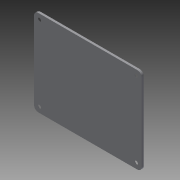
# Autodesk Inventor part: WYKONAWCY
Saved by Autodesk Inventor 2014 (Build 180170000, 170)
## iProperties
Created: 2017-04-20
Part Number: WYKONAWCY
Material: Ogólny
Document SubType Name: Modeling
Designer: hpdc7700
Density: 1 g/cm^3
Appearance: Domyślna
Author: hpdc7700
Autodesk Inventor part; units mm, degrees
(part 1 of 3)
ref_plane "YZ Plane" through (0, 0, 0) normal (1, 0, 0) x (0, 1, 0)
ref_plane "XZ Plane" through (0, 0, 0) normal (0, 1, 0) x (-1, 0, 0)
ref_plane "XY Plane" through (0, 0, 0) normal (0, 0, 1) x (1, 0, 0)
sketch "Szkic1" plane through (0, 0, 0) normal (0, 1, 0) x (-1, 0, 0)
  line L0 (-50, -40) -> (50, -40)
  line L1 (50, -40) -> (50, 40)
  line L2 (50, 40) -> (-50, 40)
  line L3 (-50, 40) -> (-50, -40)
  line L4 (-50, -40) -> (50, 40) construction
  line L5 (50, -40) -> (-50, 40) construction
  point P0 (0, 0)
  dimension "d0" = 100
  dimension "d1" = 80
  constraints: 12 end point, 2 midpoint, 2 parallel, 1 horizontal, 1 perpendicular
  measures "d0" distance of L2.end L1.end
  measures "d1" distance of L1.end L0.end
extrude "Wyciągnięcie proste1" add sketch "Szkic1" along normal blind 2
sketch "Szkic2" plane through (0, 2, 0) normal (0, 1, 0) x (1, 0, 0)
  line L0 (-46.7747, 36.4699) -> (46.5954, 36.4699) construction
  line L1 (46.5954, 36.4699) -> (46.5954, -36.8283) construction
  line L2 (46.5954, -36.8283) -> (-46.7747, -36.8283) construction
  line L3 (-46.7747, -36.8283) -> (-46.7747, 36.4699) construction
  line L4 (-33.4162, 27.0179) -> (-34.6723, 22.0179)
  line L5 (-34.6723, 22.0179) -> (-35.4178, 22.0179)
  line L6 (-35.4178, 22.0179) -> (-36.4348, 26.167)
  line L7 (-36.4348, 26.167) -> (-37.4235, 22.0179)
  line L8 (-37.4235, 22.0179) -> (-38.1609, 22.0179)
  line L9 (-38.1609, 22.0179) -> (-39.4373, 27.0179)
  line L10 (-39.4373, 27.0179) -> (-38.7525, 27.0179)
  line L11 (-38.7525, 27.0179) -> (-37.7476, 22.8728)
  line L12 (-37.7476, 22.8728) -> (-36.7509, 27.0179)
  line L13 (-36.7509, 27.0179) -> (-36.0742, 27.0179)
  line L14 (-36.0742, 27.0179) -> (-35.0693, 22.8242)
  line L15 (-35.0693, 22.8242) -> (-34.0685, 27.0179)
  line L16 (-34.0685, 27.0179) -> (-33.4162, 27.0179)
  line L17 (-29.3198, 27.0179) -> (-31.0094, 24.2302)
  line L18 (-31.0094, 24.2302) -> (-31.0094, 22.0179)
  line L19 (-31.0094, 22.0179) -> (-31.6739, 22.0179)
  line L20 (-31.6739, 22.0179) -> (-31.6739, 24.1613)
  line L21 (-31.6739, 24.1613) -> (-33.3635, 27.0179)
  line L22 (-33.3635, 27.0179) -> (-32.6261, 27.0179)
  line L23 (-32.6261, 27.0179) -> (-31.3376, 24.8177)
  line L24 (-31.3376, 24.8177) -> (-30.0248, 27.0179)
  line L25 (-30.0248, 27.0179) -> (-29.3198, 27.0179)
  line L26 (-25.2112, 22.0179) -> (-26.0742, 22.0179)
  line L27 (-26.0742, 22.0179) -> (-27.9016, 24.3437)
  line L28 (-27.9016, 24.3437) -> (-28.1933, 24.0155)
  line L29 (-28.1933, 24.0155) -> (-28.1933, 22.0179)
  line L30 (-28.1933, 22.0179) -> (-28.8578, 22.0179)
  line L31 (-28.8578, 22.0179) -> (-28.8578, 27.0179)
  line L32 (-28.8578, 27.0179) -> (-28.1933, 27.0179)
  line L33 (-28.1933, 27.0179) -> (-28.1933, 24.7205)
  line L34 (-28.1933, 24.7205) -> (-26.1431, 27.0179)
  line L35 (-26.1431, 27.0179) -> (-25.3327, 27.0179)
  line L36 (-25.3327, 27.0179) -> (-27.4032, 24.7853)
  line L37 (-27.4032, 24.7853) -> (-25.2112, 22.0179)
  spline S0 degree 2 poles (-21.2768, 26.4466) (-20.9932, 26.1143) (-20.6771, 25.1419) (-20.6771, 24.5179) knots 0 0 0 1 2 2 2
  spline S1 degree 2 poles (-20.6771, 24.5179) (-20.6771, 23.9101) (-20.9851, 22.9255) (-21.2768, 22.5933) knots 0 0 0 1 2 2 2
  spline S2 degree 2 poles (-21.2768, 22.5933) (-21.5847, 22.2448) (-22.3992, 21.9125) (-22.8894, 21.9125) knots 0 0 0 1 2 2 2
  spline S3 degree 2 poles (-22.8894, 21.9125) (-23.3959, 21.9125) (-24.2063, 22.257) (-24.5021, 22.5933) knots 0 0 0 1 2 2 2
  spline S4 degree 2 poles (-24.5021, 22.5933) (-24.7898, 22.9255) (-25.0977, 23.902) (-25.0977, 24.5179) knots 0 0 0 1 2 2 2
  spline S5 degree 2 poles (-25.0977, 24.5179) (-25.0977, 25.1459) (-24.7857, 26.1022) (-24.498, 26.4466) knots 0 0 0 1 2 2 2
  spline S6 degree 2 poles (-24.498, 26.4466) (-24.2063, 26.7788) (-23.3919, 27.1232) (-22.8894, 27.1232) knots 0 0 0 1 2 2 2
  spline S7 degree 2 poles (-22.8894, 27.1232) (-22.3789, 27.1232) (-21.5604, 26.7667) (-21.2768, 26.4466) knots 0 0 0 1 2 2 2
  spline S8 degree 2 poles (-21.37, 24.5179) (-21.37, 25.0122) (-21.5847, 25.778) (-21.7792, 26.0292) knots 0 0 0 1 2 2 2
  spline S9 degree 2 poles (-21.7792, 26.0292) (-21.9778, 26.2886) (-22.5369, 26.5479) (-22.8854, 26.5479) knots 0 0 0 1 2 2 2
  spline S10 degree 2 poles (-22.8854, 26.5479) (-23.246, 26.5479) (-23.789, 26.2967) (-23.9956, 26.0292) knots 0 0 0 1 2 2 2
  spline S11 degree 2 poles (-23.9956, 26.0292) (-24.1941, 25.774) (-24.4048, 25.0041) (-24.4048, 24.5179) knots 0 0 0 1 2 2 2
  spline S12 degree 2 poles (-24.4048, 24.5179) (-24.4048, 23.5333) (-23.5783, 22.4879) (-22.8854, 22.4879) knots 0 0 0 1 2 2 2
  spline S13 degree 2 poles (-22.8854, 22.4879) (-22.1925, 22.4879) (-21.37, 23.5333) (-21.37, 24.5179) knots 0 0 0 1 2 2 2
  line L38 (-16.37, 22.0179) -> (-17.1155, 22.0179)
  line L39 (-17.1155, 22.0179) -> (-19.3279, 26.3291)
  line L40 (-19.3279, 26.3291) -> (-19.3279, 22.0179)
  line L41 (-19.3279, 22.0179) -> (-19.9478, 22.0179)
  line L42 (-19.9478, 22.0179) -> (-19.9478, 27.0179)
  line L43 (-19.9478, 27.0179) -> (-19.0037, 27.0179)
  line L44 (-19.0037, 27.0179) -> (-16.9899, 23.0592)
  line L45 (-16.9899, 23.0592) -> (-16.9899, 27.0179)
  line L46 (-16.9899, 27.0179) -> (-16.37, 27.0179)
  line L47 (-16.37, 27.0179) -> (-16.37, 22.0179)
  line L48 (-15.8959, 22.0179) -> (-14.2104, 27.0179)
  line L49 (-14.2104, 27.0179) -> (-13.3919, 27.0179)
  line L50 (-13.3919, 27.0179) -> (-11.7063, 22.0179)
  line L51 (-11.7063, 22.0179) -> (-12.4073, 22.0179)
  line L52 (-12.4073, 22.0179) -> (-12.8611, 23.4158)
  line L53 (-12.8611, 23.4158) -> (-14.7695, 23.4158)
  line L54 (-14.7695, 23.4158) -> (-15.2233, 22.0179)
  line L55 (-15.2233, 22.0179) -> (-15.8959, 22.0179)
  line L56 (-13.0434, 23.983) -> (-13.8173, 26.3372)
  line L57 (-13.8173, 26.3372) -> (-14.5872, 23.983)
  line L58 (-14.5872, 23.983) -> (-13.0434, 23.983)
  line L59 (-5.6285, 27.0179) -> (-6.8846, 22.0179)
  line L60 (-6.8846, 22.0179) -> (-7.6301, 22.0179)
  line L61 (-7.6301, 22.0179) -> (-8.6471, 26.167)
  line L62 (-8.6471, 26.167) -> (-9.6358, 22.0179)
  line L63 (-9.6358, 22.0179) -> (-10.3732, 22.0179)
  line L64 (-10.3732, 22.0179) -> (-11.6496, 27.0179)
  line L65 (-11.6496, 27.0179) -> (-10.9648, 27.0179)
  line L66 (-10.9648, 27.0179) -> (-9.9599, 22.8728)
  line L67 (-9.9599, 22.8728) -> (-8.9632, 27.0179)
  line L68 (-8.9632, 27.0179) -> (-8.2865, 27.0179)
  line L69 (-8.2865, 27.0179) -> (-7.2817, 22.8242)
  line L70 (-7.2817, 22.8242) -> (-6.2809, 27.0179)
  line L71 (-6.2809, 27.0179) -> (-5.6285, 27.0179)
  spline S14 degree 2 poles (-3.0799, 21.9288) (-3.5661, 21.9288) (-4.3886, 22.257) (-4.6885, 22.5852) knots 0 0 0 1 2 2 2
  spline S15 degree 2 poles (-4.6885, 22.5852) (-4.9883, 22.9093) (-5.3165, 23.8817) (-5.3165, 24.5138) knots 0 0 0 1 2 2 2
  spline S16 degree 2 poles (-5.3165, 24.5138) (-5.3165, 25.1419) (-4.9964, 26.0738) (-4.6925, 26.4182) knots 0 0 0 1 2 2 2
  spline S17 degree 2 poles (-4.6925, 26.4182) (-4.3927, 26.7545) (-3.5742, 27.107) (-3.0677, 27.107) knots 0 0 0 1 2 2 2
  spline S18 degree 2 poles (-3.0677, 27.107) (-2.8165, 27.107) (-2.3749, 27.0341) (-2.1885, 26.9774) knots 0 0 0 1 2 2 2
  spline S19 degree 2 poles (-2.1885, 26.9774) (-2.0264, 26.9247) (-1.6901, 26.7748) (-1.524, 26.6856) knots 0 0 0 1 2 2 2
  line L72 (-1.524, 26.6856) -> (-1.524, 25.8834)
  line L73 (-1.524, 25.8834) -> (-1.5766, 25.8834)
  spline S20 degree 2 poles (-1.5766, 25.8834) (-1.6658, 25.9644) (-1.9413, 26.1913) (-2.1398, 26.3007) knots 0 0 0 1 2 2 2
  spline S21 degree 2 poles (-2.1398, 26.3007) (-2.3303, 26.4061) (-2.78, 26.5398) (-3.0718, 26.5398) knots 0 0 0 1 2 2 2
  spline S22 degree 2 poles (-3.0718, 26.5398) (-3.3919, 26.5398) (-3.9632, 26.2764) (-4.1779, 26.0252) knots 0 0 0 1 2 2 2
  spline S23 degree 2 poles (-4.1779, 26.0252) (-4.3886, 25.7699) (-4.6236, 24.996) (-4.6236, 24.5138) knots 0 0 0 1 2 2 2
  spline S24 degree 2 poles (-4.6236, 24.5138) (-4.6236, 23.9993) (-4.3765, 23.2578) (-4.1617, 23.0025) knots 0 0 0 1 2 2 2
  spline S25 degree 2 poles (-4.1617, 23.0025) (-3.951, 22.7553) (-3.3878, 22.5041) (-3.0718, 22.5041) knots 0 0 0 1 2 2 2
  spline S26 degree 2 poles (-3.0718, 22.5041) (-2.7841, 22.5041) (-2.2938, 22.6459) (-2.1034, 22.7513) knots 0 0 0 1 2 2 2
  spline S27 degree 2 poles (-2.1034, 22.7513) (-1.921, 22.8566) (-1.6496, 23.0754) (-1.5726, 23.1524) knots 0 0 0 1 2 2 2
  line L74 (-1.5726, 23.1524) -> (-1.524, 23.1524)
  line L75 (-1.524, 23.1524) -> (-1.524, 22.3582)
  spline S28 degree 2 poles (-1.524, 22.3582) (-1.6901, 22.2813) (-1.9818, 22.1394) (-2.1885, 22.0746) knots 0 0 0 1 2 2 2
  spline S29 degree 2 poles (-2.1885, 22.0746) (-2.4073, 22.0017) (-2.78, 21.9288) (-3.0799, 21.9288) knots 0 0 0 1 2 2 2
  line L76 (2.5968, 27.0179) -> (0.9072, 24.2302)
  line L77 (0.9072, 24.2302) -> (0.9072, 22.0179)
  line L78 (0.9072, 22.0179) -> (0.2426, 22.0179)
  line L79 (0.2426, 22.0179) -> (0.2426, 24.1613)
  line L80 (0.2426, 24.1613) -> (-1.447, 27.0179)
  line L81 (-1.447, 27.0179) -> (-0.7095, 27.0179)
  line L82 (-0.7095, 27.0179) -> (0.579, 24.8177)
  line L83 (0.579, 24.8177) -> (1.8918, 27.0179)
  line L84 (1.8918, 27.0179) -> (2.5968, 27.0179)
  spline S30 degree 2 poles (8.3666, 25.5106) (8.3666, 25.1864) (8.1357, 24.603) (7.929, 24.4004) knots 0 0 0 1 2 2 2
  spline S31 degree 2 poles (7.929, 24.4004) (7.6697, 24.1451) (6.9687, 23.8817) (6.4339, 23.8817) knots 0 0 0 1 2 2 2
  line L85 (6.4339, 23.8817) -> (5.8707, 23.8817)
  line L86 (5.8707, 23.8817) -> (5.8707, 22.0179)
  line L87 (5.8707, 22.0179) -> (5.2062, 22.0179)
  line L88 (5.2062, 22.0179) -> (5.2062, 27.0179)
  line L89 (5.2062, 27.0179) -> (6.4623, 27.0179)
  spline S32 degree 2 poles (6.4623, 27.0179) (6.908, 27.0179) (7.5319, 26.872) (7.771, 26.7059) knots 0 0 0 1 2 2 2
  spline S33 degree 2 poles (7.771, 26.7059) (8.0506, 26.5155) (8.3666, 25.9279) (8.3666, 25.5106) knots 0 0 0 1 2 2 2
  spline S34 degree 2 poles (7.6738, 25.4903) (7.6738, 25.7497) (7.4955, 26.1305) (7.3131, 26.2521) knots 0 0 0 1 2 2 2
  spline S35 degree 2 poles (7.3131, 26.2521) (7.1551, 26.3574) (6.7337, 26.4425) (6.4217, 26.4425) knots 0 0 0 1 2 2 2
  line L90 (6.4217, 26.4425) -> (5.8707, 26.4425)
  line L91 (5.8707, 26.4425) -> (5.8707, 24.449)
  line L92 (5.8707, 24.449) -> (6.3245, 24.449)
  spline S36 degree 2 poles (6.3245, 24.449) (6.7297, 24.449) (7.2281, 24.5787) (7.3901, 24.7488) knots 0 0 0 1 2 2 2
  spline S37 degree 2 poles (7.3901, 24.7488) (7.5401, 24.8988) (7.6738, 25.2513) (7.6738, 25.4903) knots 0 0 0 1 2 2 2
  line L93 (12.8683, 22.0179) -> (12.0052, 22.0179)
  line L94 (12.0052, 22.0179) -> (10.425, 24.0074)
  line L95 (10.425, 24.0074) -> (9.6632, 24.0074)
  line L96 (9.6632, 24.0074) -> (9.6632, 22.0179)
  line L97 (9.6632, 22.0179) -> (8.9987, 22.0179)
  line L98 (8.9987, 22.0179) -> (8.9987, 27.0179)
  line L99 (8.9987, 27.0179) -> (10.2872, 27.0179)
  spline S38 degree 2 poles (10.2872, 27.0179) (10.7167, 27.0179) (11.2961, 26.9247) (11.5595, 26.7545) knots 0 0 0 1 2 2 2
  spline S39 degree 2 poles (11.5595, 26.7545) (11.8229, 26.5843) (12.1268, 26.0535) (12.1268, 25.6605) knots 0 0 0 1 2 2 2
  spline S40 degree 2 poles (12.1268, 25.6605) (12.1268, 25.1135) (11.5676, 24.372) (11.0895, 24.1937) knots 0 0 0 1 2 2 2
  line L100 (11.0895, 24.1937) -> (12.8683, 22.0179)
  spline S41 degree 2 poles (11.4339, 25.6078) (11.4339, 25.8266) (11.2799, 26.1629) (11.1178, 26.2723) knots 0 0 0 1 2 2 2
  spline S42 degree 2 poles (11.1178, 26.2723) (10.976, 26.3655) (10.5992, 26.4425) (10.3237, 26.4425) knots 0 0 0 1 2 2 2
  line L101 (10.3237, 26.4425) -> (9.6632, 26.4425)
  line L102 (9.6632, 26.4425) -> (9.6632, 24.5625)
  line L103 (9.6632, 24.5625) -> (10.2467, 24.5625)
  spline S43 degree 2 poles (10.2467, 24.5625) (10.5344, 24.5625) (10.9922, 24.6638) (11.1503, 24.8218) knots 0 0 0 1 2 2 2
  spline S44 degree 2 poles (11.1503, 24.8218) (11.2961, 24.9595) (11.4339, 25.3485) (11.4339, 25.6078) knots 0 0 0 1 2 2 2
  spline S45 degree 2 poles (16.8026, 26.4466) (17.0862, 26.1143) (17.4023, 25.1419) (17.4023, 24.5179) knots 0 0 0 1 2 2 2
  spline S46 degree 2 poles (17.4023, 24.5179) (17.4023, 23.9101) (17.0943, 22.9255) (16.8026, 22.5933) knots 0 0 0 1 2 2 2
  spline S47 degree 2 poles (16.8026, 22.5933) (16.4947, 22.2448) (15.6802, 21.9125) (15.19, 21.9125) knots 0 0 0 1 2 2 2
  spline S48 degree 2 poles (15.19, 21.9125) (14.6835, 21.9125) (13.8731, 22.257) (13.5773, 22.5933) knots 0 0 0 1 2 2 2
  spline S49 degree 2 poles (13.5773, 22.5933) (13.2896, 22.9255) (12.9817, 23.902) (12.9817, 24.5179) knots 0 0 0 1 2 2 2
  spline S50 degree 2 poles (12.9817, 24.5179) (12.9817, 25.1459) (13.2937, 26.1022) (13.5814, 26.4466) knots 0 0 0 1 2 2 2
  spline S51 degree 2 poles (13.5814, 26.4466) (13.8731, 26.7788) (14.6875, 27.1232) (15.19, 27.1232) knots 0 0 0 1 2 2 2
  spline S52 degree 2 poles (15.19, 27.1232) (15.7005, 27.1232) (16.519, 26.7667) (16.8026, 26.4466) knots 0 0 0 1 2 2 2
  spline S53 degree 2 poles (16.7094, 24.5179) (16.7094, 25.0122) (16.4947, 25.778) (16.3002, 26.0292) knots 0 0 0 1 2 2 2
  spline S54 degree 2 poles (16.3002, 26.0292) (16.1016, 26.2886) (15.5425, 26.5479) (15.194, 26.5479) knots 0 0 0 1 2 2 2
  spline S55 degree 2 poles (15.194, 26.5479) (14.8334, 26.5479) (14.2905, 26.2967) (14.0838, 26.0292) knots 0 0 0 1 2 2 2
  spline S56 degree 2 poles (14.0838, 26.0292) (13.8853, 25.774) (13.6746, 25.0041) (13.6746, 24.5179) knots 0 0 0 1 2 2 2
  spline S57 degree 2 poles (13.6746, 24.5179) (13.6746, 23.5333) (14.5012, 22.4879) (15.194, 22.4879) knots 0 0 0 1 2 2 2
  spline S58 degree 2 poles (15.194, 22.4879) (15.8869, 22.4879) (16.7094, 23.5333) (16.7094, 24.5179) knots 0 0 0 1 2 2 2
  spline S59 degree 2 poles (20.0157, 23.3185) (20.0157, 22.6621) (19.2135, 21.949) (18.5368, 21.949) knots 0 0 0 1 2 2 2
  spline S60 degree 2 poles (18.5368, 21.949) (18.3747, 21.949) (17.8358, 22.0057) (17.6535, 22.0463) knots 0 0 0 1 2 2 2
  line L104 (17.6535, 22.0463) -> (17.6535, 22.6864)
  line L105 (17.6535, 22.6864) -> (17.69, 22.6864)
  spline S61 degree 2 poles (17.69, 22.6864) (17.8277, 22.6378) (18.237, 22.5244) (18.4477, 22.5244) knots 0 0 0 1 2 2 2
  spline S62 degree 2 poles (18.4477, 22.5244) (18.7556, 22.5244) (19.1243, 22.6662) (19.2094, 22.7958) knots 0 0 0 1 2 2 2
  spline S63 degree 2 poles (19.2094, 22.7958) (19.3026, 22.9296) (19.3512, 23.3185) (19.3512, 23.5738) knots 0 0 0 1 2 2 2
  line L106 (19.3512, 23.5738) -> (19.3512, 26.4871)
  line L107 (19.3512, 26.4871) -> (18.2937, 26.4871)
  line L108 (18.2937, 26.4871) -> (18.2937, 27.0179)
  line L109 (18.2937, 27.0179) -> (20.0157, 27.0179)
  line L110 (20.0157, 27.0179) -> (20.0157, 23.3185)
  line L111 (20.9963, 22.0179) -> (20.9963, 27.0179)
  line L112 (20.9963, 27.0179) -> (24.1243, 27.0179)
  line L113 (24.1243, 27.0179) -> (24.1243, 26.4263)
  line L114 (24.1243, 26.4263) -> (21.6608, 26.4263)
  line L115 (21.6608, 26.4263) -> (21.6608, 25.0568)
  line L116 (21.6608, 25.0568) -> (23.9582, 25.0568)
  line L117 (23.9582, 25.0568) -> (23.9582, 24.4652)
  line L118 (23.9582, 24.4652) -> (21.6608, 24.4652)
  line L119 (21.6608, 24.4652) -> (21.6608, 22.6095)
  line L120 (21.6608, 22.6095) -> (24.1243, 22.6095)
  line L121 (24.1243, 22.6095) -> (24.1243, 22.0179)
  line L122 (24.1243, 22.0179) -> (20.9963, 22.0179)
  line L123 (28.5003, 22.0179) -> (27.6373, 22.0179)
  line L124 (27.6373, 22.0179) -> (25.8099, 24.3437)
  line L125 (25.8099, 24.3437) -> (25.5182, 24.0155)
  line L126 (25.5182, 24.0155) -> (25.5182, 22.0179)
  line L127 (25.5182, 22.0179) -> (24.8537, 22.0179)
  line L128 (24.8537, 22.0179) -> (24.8537, 27.0179)
  line L129 (24.8537, 27.0179) -> (25.5182, 27.0179)
  line L130 (25.5182, 27.0179) -> (25.5182, 24.7205)
  line L131 (25.5182, 24.7205) -> (27.5684, 27.0179)
  line L132 (27.5684, 27.0179) -> (28.3788, 27.0179)
  line L133 (28.3788, 27.0179) -> (26.3083, 24.7853)
  line L134 (26.3083, 24.7853) -> (28.5003, 22.0179)
  line L135 (30.0644, 22.0179) -> (30.0644, 26.4263)
  line L136 (30.0644, 26.4263) -> (28.3869, 26.4263)
  line L137 (28.3869, 26.4263) -> (28.3869, 27.0179)
  line L138 (28.3869, 27.0179) -> (32.4063, 27.0179)
  line L139 (32.4063, 27.0179) -> (32.4063, 26.4263)
  line L140 (32.4063, 26.4263) -> (30.7289, 26.4263)
  line L141 (30.7289, 26.4263) -> (30.7289, 22.0179)
  line L142 (30.7289, 22.0179) -> (30.0644, 22.0179)
  spline S64 degree 2 poles (34.6592, 21.9125) (34.2175, 21.9125) (33.5611, 22.1435) (33.3302, 22.3745) knots 0 0 0 1 2 2 2
  spline S65 degree 2 poles (33.3302, 22.3745) (33.0668, 22.6338) (32.852, 23.3631) (32.852, 23.898) knots 0 0 0 1 2 2 2
  line L143 (32.852, 23.898) -> (32.852, 27.0179)
  line L144 (32.852, 27.0179) -> (33.5166, 27.0179)
  line L145 (33.5166, 27.0179) -> (33.5166, 23.898)
  spline S66 degree 2 poles (33.5166, 23.898) (33.5166, 23.5495) (33.6057, 23.0795) (33.7313, 22.889) knots 0 0 0 1 2 2 2
  spline S67 degree 2 poles (33.7313, 22.889) (33.865, 22.6864) (34.3269, 22.4798) (34.6592, 22.4798) knots 0 0 0 1 2 2 2
  spline S68 degree 2 poles (34.6592, 22.4798) (34.9712, 22.4798) (35.4574, 22.6864) (35.5911, 22.889) knots 0 0 0 1 2 2 2
  spline S69 degree 2 poles (35.5911, 22.889) (35.7167, 23.0795) (35.8059, 23.5454) (35.8059, 23.8817) knots 0 0 0 1 2 2 2
  line L146 (35.8059, 23.8817) -> (35.8059, 27.0179)
  line L147 (35.8059, 27.0179) -> (36.4704, 27.0179)
  line L148 (36.4704, 27.0179) -> (36.4704, 23.898)
  spline S70 degree 2 poles (36.4704, 23.898) (36.4704, 23.3753) (36.2597, 22.6297) (35.9922, 22.3745) knots 0 0 0 1 2 2 2
  spline S71 degree 2 poles (35.9922, 22.3745) (35.7532, 22.1394) (35.1211, 21.9125) (34.6592, 21.9125) knots 0 0 0 1 2 2 2
  line L149 (38.5328, 22.0179) -> (37.7305, 22.0179)
  line L150 (37.7305, 22.0179) -> (37.7305, 22.9741)
  line L151 (37.7305, 22.9741) -> (38.5328, 22.9741)
  line L152 (38.5328, 22.9741) -> (38.5328, 22.0179)
  line L153 (38.5328, 24.8137) -> (37.7305, 24.8137)
  line L154 (37.7305, 24.8137) -> (37.7305, 25.7699)
  line L155 (37.7305, 25.7699) -> (38.5328, 25.7699)
  line L156 (38.5328, 25.7699) -> (38.5328, 24.8137)
  spline S72 degree 2 poles (-26.7792, 15.0862) (-26.7792, 14.4298) (-27.5815, 13.7166) (-28.2582, 13.7166) knots 0 0 0 1 2 2 2
  spline S73 degree 2 poles (-28.2582, 13.7166) (-28.4202, 13.7166) (-28.9591, 13.7734) (-29.1415, 13.8139) knots 0 0 0 1 2 2 2
  line L157 (-29.1415, 13.8139) -> (-29.1415, 14.4541)
  line L158 (-29.1415, 14.4541) -> (-29.105, 14.4541)
  spline S74 degree 2 poles (-29.105, 14.4541) (-28.9672, 14.4055) (-28.558, 14.292) (-28.3473, 14.292) knots 0 0 0 1 2 2 2
  spline S75 degree 2 poles (-28.3473, 14.292) (-28.0394, 14.292) (-27.6706, 14.4338) (-27.5856, 14.5635) knots 0 0 0 1 2 2 2
  spline S76 degree 2 poles (-27.5856, 14.5635) (-27.4924, 14.6972) (-27.4437, 15.0862) (-27.4437, 15.3414) knots 0 0 0 1 2 2 2
  line L159 (-27.4437, 15.3414) -> (-27.4437, 18.2547)
  line L160 (-27.4437, 18.2547) -> (-28.5013, 18.2547)
  line L161 (-28.5013, 18.2547) -> (-28.5013, 18.7855)
  line L162 (-28.5013, 18.7855) -> (-26.7792, 18.7855)
  line L163 (-26.7792, 18.7855) -> (-26.7792, 15.0862)
  line L164 (-26.3376, 13.7855) -> (-24.652, 18.7855)
  line L165 (-24.652, 18.7855) -> (-23.8335, 18.7855)
  line L166 (-23.8335, 18.7855) -> (-22.148, 13.7855)
  line L167 (-22.148, 13.7855) -> (-22.8489, 13.7855)
  line L168 (-22.8489, 13.7855) -> (-23.3027, 15.1834)
  line L169 (-23.3027, 15.1834) -> (-25.2112, 15.1834)
  line L170 (-25.2112, 15.1834) -> (-25.665, 13.7855)
  line L171 (-25.665, 13.7855) -> (-26.3376, 13.7855)
  line L172 (-23.4851, 15.7507) -> (-24.259, 18.1048)
  line L173 (-24.259, 18.1048) -> (-25.0288, 15.7507)
  line L174 (-25.0288, 15.7507) -> (-23.4851, 15.7507)
  spline S77 degree 2 poles (-19.7209, 13.6964) (-20.2071, 13.6964) (-21.0296, 14.0246) (-21.3295, 14.3528) knots 0 0 0 1 2 2 2
  spline S78 degree 2 poles (-21.3295, 14.3528) (-21.6293, 14.6769) (-21.9575, 15.6494) (-21.9575, 16.2815) knots 0 0 0 1 2 2 2
  spline S79 degree 2 poles (-21.9575, 16.2815) (-21.9575, 16.9095) (-21.6374, 17.8414) (-21.3335, 18.1858) knots 0 0 0 1 2 2 2
  spline S80 degree 2 poles (-21.3335, 18.1858) (-21.0337, 18.5222) (-20.2152, 18.8747) (-19.7087, 18.8747) knots 0 0 0 1 2 2 2
  spline S81 degree 2 poles (-19.7087, 18.8747) (-19.4575, 18.8747) (-19.0159, 18.8017) (-18.8295, 18.745) knots 0 0 0 1 2 2 2
  spline S82 degree 2 poles (-18.8295, 18.745) (-18.6674, 18.6923) (-18.3311, 18.5424) (-18.165, 18.4533) knots 0 0 0 1 2 2 2
  line L175 (-18.165, 18.4533) -> (-18.165, 17.651)
  line L176 (-18.165, 17.651) -> (-18.2176, 17.651)
  spline S83 degree 2 poles (-18.2176, 17.651) (-18.3068, 17.732) (-18.5823, 17.9589) (-18.7809, 18.0683) knots 0 0 0 1 2 2 2
  spline S84 degree 2 poles (-18.7809, 18.0683) (-18.9713, 18.1737) (-19.421, 18.3074) (-19.7128, 18.3074) knots 0 0 0 1 2 2 2
  spline S85 degree 2 poles (-19.7128, 18.3074) (-20.0329, 18.3074) (-20.6042, 18.044) (-20.8189, 17.7928) knots 0 0 0 1 2 2 2
  spline S86 degree 2 poles (-20.8189, 17.7928) (-21.0296, 17.5375) (-21.2646, 16.7636) (-21.2646, 16.2815) knots 0 0 0 1 2 2 2
  spline S87 degree 2 poles (-21.2646, 16.2815) (-21.2646, 15.7669) (-21.0175, 15.0254) (-20.8027, 14.7701) knots 0 0 0 1 2 2 2
  spline S88 degree 2 poles (-20.8027, 14.7701) (-20.592, 14.523) (-20.0288, 14.2717) (-19.7128, 14.2717) knots 0 0 0 1 2 2 2
  spline S89 degree 2 poles (-19.7128, 14.2717) (-19.4251, 14.2717) (-18.9348, 14.4136) (-18.7444, 14.5189) knots 0 0 0 1 2 2 2
  spline S90 degree 2 poles (-18.7444, 14.5189) (-18.5621, 14.6243) (-18.2906, 14.8431) (-18.2136, 14.92) knots 0 0 0 1 2 2 2
  line L177 (-18.2136, 14.92) -> (-18.165, 14.92)
  line L178 (-18.165, 14.92) -> (-18.165, 14.1259)
  spline S91 degree 2 poles (-18.165, 14.1259) (-18.3311, 14.0489) (-18.6228, 13.9071) (-18.8295, 13.8422) knots 0 0 0 1 2 2 2
  spline S92 degree 2 poles (-18.8295, 13.8422) (-19.0483, 13.7693) (-19.421, 13.6964) (-19.7209, 13.6964) knots 0 0 0 1 2 2 2
  line L179 (-17.545, 13.7855) -> (-17.545, 18.7855)
  line L180 (-17.545, 18.7855) -> (-14.417, 18.7855)
  line L181 (-14.417, 18.7855) -> (-14.417, 18.194)
  line L182 (-14.417, 18.194) -> (-16.8805, 18.194)
  line L183 (-16.8805, 18.194) -> (-16.8805, 16.8244)
  line L184 (-16.8805, 16.8244) -> (-14.5831, 16.8244)
  line L185 (-14.5831, 16.8244) -> (-14.5831, 16.2328)
  line L186 (-14.5831, 16.2328) -> (-16.8805, 16.2328)
  line L187 (-16.8805, 16.2328) -> (-16.8805, 14.3771)
  line L188 (-16.8805, 14.3771) -> (-14.417, 14.3771)
  line L189 (-14.417, 14.3771) -> (-14.417, 13.7855)
  line L190 (-14.417, 13.7855) -> (-17.545, 13.7855)
  line L191 (-10.041, 13.7855) -> (-10.904, 13.7855)
  line L192 (-10.904, 13.7855) -> (-12.7314, 16.1113)
  line L193 (-12.7314, 16.1113) -> (-13.0232, 15.7831)
  line L194 (-13.0232, 15.7831) -> (-13.0232, 13.7855)
  line L195 (-13.0232, 13.7855) -> (-13.6877, 13.7855)
  line L196 (-13.6877, 13.7855) -> (-13.6877, 18.7855)
  line L197 (-13.6877, 18.7855) -> (-13.0232, 18.7855)
  line L198 (-13.0232, 18.7855) -> (-13.0232, 16.4881)
  line L199 (-13.0232, 16.4881) -> (-10.9729, 18.7855)
  line L200 (-10.9729, 18.7855) -> (-10.1625, 18.7855)
  line L201 (-10.1625, 18.7855) -> (-12.233, 16.5529)
  line L202 (-12.233, 16.5529) -> (-10.041, 13.7855)
  line L203 (-3.2095, 13.7855) -> (-3.874, 13.7855)
  line L204 (-3.874, 13.7855) -> (-3.874, 18.0927)
  line L205 (-3.874, 18.0927) -> (-5.1787, 15.1632)
  line L206 (-5.1787, 15.1632) -> (-5.5839, 15.1632)
  line L207 (-5.5839, 15.1632) -> (-6.8765, 18.0927)
  line L208 (-6.8765, 18.0927) -> (-6.8765, 13.7855)
  line L209 (-6.8765, 13.7855) -> (-7.4964, 13.7855)
  line L210 (-7.4964, 13.7855) -> (-7.4964, 18.7855)
  line L211 (-7.4964, 18.7855) -> (-6.5888, 18.7855)
  line L212 (-6.5888, 18.7855) -> (-5.3408, 16.0019)
  line L213 (-5.3408, 16.0019) -> (-4.1334, 18.7855)
  line L214 (-4.1334, 18.7855) -> (-3.2095, 18.7855)
  line L215 (-3.2095, 18.7855) -> (-3.2095, 13.7855)
  line L216 (-2.7355, 13.7855) -> (-1.0499, 18.7855)
  line L217 (-1.0499, 18.7855) -> (-0.2314, 18.7855)
  line L218 (-0.2314, 18.7855) -> (1.4542, 13.7855)
  line L219 (1.4542, 13.7855) -> (0.7532, 13.7855)
  line L220 (0.7532, 13.7855) -> (0.2994, 15.1834)
  line L221 (0.2994, 15.1834) -> (-1.6091, 15.1834)
  line L222 (-1.6091, 15.1834) -> (-2.0629, 13.7855)
  line L223 (-2.0629, 13.7855) -> (-2.7355, 13.7855)
  line L224 (0.117, 15.7507) -> (-0.6569, 18.1048)
  line L225 (-0.6569, 18.1048) -> (-1.4267, 15.7507)
  line L226 (-1.4267, 15.7507) -> (0.117, 15.7507)
  line L227 (5.7978, 13.7855) -> (4.9347, 13.7855)
  line L228 (4.9347, 13.7855) -> (3.3545, 15.775)
  line L229 (3.3545, 15.775) -> (2.5927, 15.775)
  line L230 (2.5927, 15.775) -> (2.5927, 13.7855)
  line L231 (2.5927, 13.7855) -> (1.9282, 13.7855)
  line L232 (1.9282, 13.7855) -> (1.9282, 18.7855)
  line L233 (1.9282, 18.7855) -> (3.2167, 18.7855)
  spline S93 degree 2 poles (3.2167, 18.7855) (3.6462, 18.7855) (4.2256, 18.6923) (4.489, 18.5222) knots 0 0 0 1 2 2 2
  spline S94 degree 2 poles (4.489, 18.5222) (4.7524, 18.352) (5.0563, 17.8212) (5.0563, 17.4281) knots 0 0 0 1 2 2 2
  spline S95 degree 2 poles (5.0563, 17.4281) (5.0563, 16.8811) (4.4971, 16.1397) (4.019, 15.9614) knots 0 0 0 1 2 2 2
  line L234 (4.019, 15.9614) -> (5.7978, 13.7855)
  spline S96 degree 2 poles (4.3634, 17.3755) (4.3634, 17.5943) (4.2094, 17.9306) (4.0473, 18.04) knots 0 0 0 1 2 2 2
  spline S97 degree 2 poles (4.0473, 18.04) (3.9055, 18.1332) (3.5287, 18.2102) (3.2532, 18.2102) knots 0 0 0 1 2 2 2
  line L235 (3.2532, 18.2102) -> (2.5927, 18.2102)
  line L236 (2.5927, 18.2102) -> (2.5927, 16.3301)
  line L237 (2.5927, 16.3301) -> (3.1762, 16.3301)
  spline S98 degree 2 poles (3.1762, 16.3301) (3.4639, 16.3301) (3.9217, 16.4314) (4.0798, 16.5894) knots 0 0 0 1 2 2 2
  spline S99 degree 2 poles (4.0798, 16.5894) (4.2256, 16.7272) (4.3634, 17.1162) (4.3634, 17.3755) knots 0 0 0 1 2 2 2
  line L238 (7.3618, 13.7855) -> (7.3618, 18.194)
  line L239 (7.3618, 18.194) -> (5.6843, 18.194)
  line L240 (5.6843, 18.194) -> (5.6843, 18.7855)
  line L241 (5.6843, 18.7855) -> (9.7037, 18.7855)
  line L242 (9.7037, 18.7855) -> (9.7037, 18.194)
  line L243 (9.7037, 18.194) -> (8.0263, 18.194)
  line L244 (8.0263, 18.194) -> (8.0263, 13.7855)
  line L245 (8.0263, 13.7855) -> (7.3618, 13.7855)
  line L246 (13.711, 18.7855) -> (12.0214, 15.9978)
  line L247 (12.0214, 15.9978) -> (12.0214, 13.7855)
  line L248 (12.0214, 13.7855) -> (11.3569, 13.7855)
  line L249 (11.3569, 13.7855) -> (11.3569, 15.929)
  line L250 (11.3569, 15.929) -> (9.6673, 18.7855)
  line L251 (9.6673, 18.7855) -> (10.4047, 18.7855)
  line L252 (10.4047, 18.7855) -> (11.6932, 16.5854)
  line L253 (11.6932, 16.5854) -> (13.006, 18.7855)
  line L254 (13.006, 18.7855) -> (13.711, 18.7855)
  line L255 (17.7508, 13.7855) -> (17.0052, 13.7855)
  line L256 (17.0052, 13.7855) -> (14.7929, 18.0967)
  line L257 (14.7929, 18.0967) -> (14.7929, 13.7855)
  line L258 (14.7929, 13.7855) -> (14.173, 13.7855)
  line L259 (14.173, 13.7855) -> (14.173, 18.7855)
  line L260 (14.173, 18.7855) -> (15.117, 18.7855)
  line L261 (15.117, 18.7855) -> (17.1308, 14.8269)
  line L262 (17.1308, 14.8269) -> (17.1308, 18.7855)
  line L263 (17.1308, 18.7855) -> (17.7508, 18.7855)
  line L264 (17.7508, 18.7855) -> (17.7508, 13.7855)
  line L265 (20.506, 13.7855) -> (18.5692, 13.7855)
  line L266 (18.5692, 13.7855) -> (18.5692, 14.2961)
  line L267 (18.5692, 14.2961) -> (19.2054, 14.2961)
  line L268 (19.2054, 14.2961) -> (19.2054, 18.275)
  line L269 (19.2054, 18.275) -> (18.5692, 18.275)
  line L270 (18.5692, 18.275) -> (18.5692, 18.7855)
  line L271 (18.5692, 18.7855) -> (20.506, 18.7855)
  line L272 (20.506, 18.7855) -> (20.506, 18.275)
  line L273 (20.506, 18.275) -> (19.8699, 18.275)
  line L274 (19.8699, 18.275) -> (19.8699, 14.2961)
  line L275 (19.8699, 14.2961) -> (20.506, 14.2961)
  line L276 (20.506, 14.2961) -> (20.506, 13.7855)
  line L277 (20.7896, 13.7855) -> (22.4752, 18.7855)
  line L278 (22.4752, 18.7855) -> (23.2937, 18.7855)
  line L279 (23.2937, 18.7855) -> (24.9793, 13.7855)
  line L280 (24.9793, 13.7855) -> (24.2783, 13.7855)
  line L281 (24.2783, 13.7855) -> (23.8245, 15.1834)
  line L282 (23.8245, 15.1834) -> (21.9161, 15.1834)
  line L283 (21.9161, 15.1834) -> (21.4623, 13.7855)
  line L284 (21.4623, 13.7855) -> (20.7896, 13.7855)
  line L285 (23.6422, 15.7507) -> (22.8683, 18.1048)
  line L286 (22.8683, 18.1048) -> (22.0984, 15.7507)
  line L287 (22.0984, 15.7507) -> (23.6422, 15.7507)
  line L288 (29.1, 13.7855) -> (28.237, 13.7855)
  line L289 (28.237, 13.7855) -> (26.4096, 16.1113)
  line L290 (26.4096, 16.1113) -> (26.1178, 15.7831)
  line L291 (26.1178, 15.7831) -> (26.1178, 13.7855)
  line L292 (26.1178, 13.7855) -> (25.4533, 13.7855)
  line L293 (25.4533, 13.7855) -> (25.4533, 18.7855)
  line L294 (25.4533, 18.7855) -> (26.1178, 18.7855)
  line L295 (26.1178, 18.7855) -> (26.1178, 16.4881)
  line L296 (26.1178, 16.4881) -> (28.1681, 18.7855)
  line L297 (28.1681, 18.7855) -> (28.9785, 18.7855)
  line L298 (28.9785, 18.7855) -> (26.908, 16.5529)
  line L299 (26.908, 16.5529) -> (29.1, 13.7855)
  line L300 (-35.2031, 5.5532) -> (-38.1001, 5.5532)
  line L301 (-38.1001, 5.5532) -> (-38.1001, 7.3765)
  line L302 (-38.1001, 7.3765) -> (-38.6633, 6.9146)
  line L303 (-38.6633, 6.9146) -> (-38.6633, 7.4494)
  line L304 (-38.6633, 7.4494) -> (-38.1001, 7.9032)
  line L305 (-38.1001, 7.9032) -> (-38.1001, 10.5532)
  line L306 (-38.1001, 10.5532) -> (-37.4356, 10.5532)
  line L307 (-37.4356, 10.5532) -> (-37.4356, 8.3814)
  line L308 (-37.4356, 8.3814) -> (-36.3376, 9.289)
  line L309 (-36.3376, 9.289) -> (-36.3376, 8.7541)
  line L310 (-36.3376, 8.7541) -> (-37.4356, 7.8627)
  line L311 (-37.4356, 7.8627) -> (-37.4356, 6.1447)
  line L312 (-37.4356, 6.1447) -> (-35.2031, 6.1447)
  line L313 (-35.2031, 6.1447) -> (-35.2031, 5.5532)
  spline S100 degree 2 poles (-32.934, 5.4478) (-33.3757, 5.4478) (-34.0321, 5.6788) (-34.263, 5.9097) knots 0 0 0 1 2 2 2
  spline S101 degree 2 poles (-34.263, 5.9097) (-34.5264, 6.169) (-34.7411, 6.8984) (-34.7411, 7.4332) knots 0 0 0 1 2 2 2
  line L314 (-34.7411, 7.4332) -> (-34.7411, 10.5532)
  line L315 (-34.7411, 10.5532) -> (-34.0766, 10.5532)
  line L316 (-34.0766, 10.5532) -> (-34.0766, 7.4332)
  spline S102 degree 2 poles (-34.0766, 7.4332) (-34.0766, 7.0848) (-33.9875, 6.6147) (-33.8619, 6.4243) knots 0 0 0 1 2 2 2
  spline S103 degree 2 poles (-33.8619, 6.4243) (-33.7282, 6.2217) (-33.2663, 6.0151) (-32.934, 6.0151) knots 0 0 0 1 2 2 2
  spline S104 degree 2 poles (-32.934, 6.0151) (-32.622, 6.0151) (-32.1358, 6.2217) (-32.0021, 6.4243) knots 0 0 0 1 2 2 2
  spline S105 degree 2 poles (-32.0021, 6.4243) (-31.8765, 6.6147) (-31.7873, 7.0807) (-31.7873, 7.417) knots 0 0 0 1 2 2 2
  line L317 (-31.7873, 7.417) -> (-31.7873, 10.5532)
  line L318 (-31.7873, 10.5532) -> (-31.1228, 10.5532)
  line L319 (-31.1228, 10.5532) -> (-31.1228, 7.4332)
  spline S106 degree 2 poles (-31.1228, 7.4332) (-31.1228, 6.9105) (-31.3335, 6.165) (-31.601, 5.9097) knots 0 0 0 1 2 2 2
  spline S107 degree 2 poles (-31.601, 5.9097) (-31.84, 5.6747) (-32.4721, 5.4478) (-32.934, 5.4478) knots 0 0 0 1 2 2 2
  line L320 (-26.524, 5.5532) -> (-27.387, 5.5532)
  line L321 (-27.387, 5.5532) -> (-29.2144, 7.8789)
  line L322 (-29.2144, 7.8789) -> (-29.5061, 7.5507)
  line L323 (-29.5061, 7.5507) -> (-29.5061, 5.5532)
  line L324 (-29.5061, 5.5532) -> (-30.1706, 5.5532)
  line L325 (-30.1706, 5.5532) -> (-30.1706, 10.5532)
  line L326 (-30.1706, 10.5532) -> (-29.5061, 10.5532)
  line L327 (-29.5061, 10.5532) -> (-29.5061, 8.2557)
  line L328 (-29.5061, 8.2557) -> (-27.4559, 10.5532)
  line L329 (-27.4559, 10.5532) -> (-26.6455, 10.5532)
  line L330 (-26.6455, 10.5532) -> (-28.716, 8.3206)
  line L331 (-28.716, 8.3206) -> (-26.524, 5.5532)
  line L332 (-26.6658, 5.5532) -> (-24.9802, 10.5532)
  line L333 (-24.9802, 10.5532) -> (-24.1617, 10.5532)
  line L334 (-24.1617, 10.5532) -> (-22.4762, 5.5532)
  line L335 (-22.4762, 5.5532) -> (-23.1771, 5.5532)
  line L336 (-23.1771, 5.5532) -> (-23.6309, 6.951)
  line L337 (-23.6309, 6.951) -> (-25.5394, 6.951)
  line L338 (-25.5394, 6.951) -> (-25.9932, 5.5532)
  line L339 (-25.9932, 5.5532) -> (-26.6658, 5.5532)
  line L340 (-23.8133, 7.5183) -> (-24.5872, 9.8724)
  line L341 (-24.5872, 9.8724) -> (-25.357, 7.5183)
  line L342 (-25.357, 7.5183) -> (-23.8133, 7.5183)
  spline S108 degree 2 poles (-20.6082, 5.464) (-21.1512, 5.464) (-21.9129, 5.6909) (-22.2492, 5.853) knots 0 0 0 1 2 2 2
  line L343 (-22.2492, 5.853) -> (-22.2492, 6.6877)
  line L344 (-22.2492, 6.6877) -> (-22.2006, 6.6877)
  spline S109 degree 2 poles (-22.2006, 6.6877) (-21.8724, 6.3797) (-21.0418, 6.0394) (-20.6569, 6.0394) knots 0 0 0 1 2 2 2
  spline S110 degree 2 poles (-20.6569, 6.0394) (-20.1058, 6.0394) (-19.5426, 6.4972) (-19.5426, 6.8741) knots 0 0 0 1 2 2 2
  spline S111 degree 2 poles (-19.5426, 6.8741) (-19.5426, 7.1739) (-19.8384, 7.5467) (-20.1585, 7.6399) knots 0 0 0 1 2 2 2
  spline S112 degree 2 poles (-20.1585, 7.6399) (-20.3894, 7.7047) (-20.7744, 7.7938) (-21.0621, 7.8668) knots 0 0 0 1 2 2 2
  spline S113 degree 2 poles (-21.0621, 7.8668) (-21.3214, 7.9357) (-21.7306, 8.1423) (-21.8886, 8.3084) knots 0 0 0 1 2 2 2
  spline S114 degree 2 poles (-21.8886, 8.3084) (-22.0426, 8.4745) (-22.2128, 8.9203) (-22.2128, 9.212) knots 0 0 0 1 2 2 2
  spline S115 degree 2 poles (-22.2128, 9.212) (-22.2128, 9.8198) (-21.2646, 10.6423) (-20.5313, 10.6423) knots 0 0 0 1 2 2 2
  spline S116 degree 2 poles (-20.5313, 10.6423) (-20.1099, 10.6423) (-19.3643, 10.4762) (-19.0442, 10.3181) knots 0 0 0 1 2 2 2
  line L345 (-19.0442, 10.3181) -> (-19.0442, 9.524)
  line L346 (-19.0442, 9.524) -> (-19.0928, 9.524)
  spline S117 degree 2 poles (-19.0928, 9.524) (-19.3319, 9.7428) (-20.0775, 10.0669) (-20.4867, 10.0669) knots 0 0 0 1 2 2 2
  spline S118 degree 2 poles (-20.4867, 10.0669) (-20.9486, 10.0669) (-21.5199, 9.6334) (-21.5199, 9.2809) knots 0 0 0 1 2 2 2
  spline S119 degree 2 poles (-21.5199, 9.2809) (-21.5199, 8.9648) (-21.1836, 8.588) (-20.8676, 8.5029) knots 0 0 0 1 2 2 2
  spline S120 degree 2 poles (-20.8676, 8.5029) (-20.6569, 8.4462) (-20.045, 8.3003) (-19.8424, 8.2395) knots 0 0 0 1 2 2 2
  spline S121 degree 2 poles (-19.8424, 8.2395) (-19.3279, 8.0815) (-18.8497, 7.4454) (-18.8497, 6.9794) knots 0 0 0 1 2 2 2
  spline S122 degree 2 poles (-18.8497, 6.9794) (-18.8497, 6.6836) (-19.0888, 6.1164) (-19.3035, 5.9178) knots 0 0 0 1 2 2 2
  spline S123 degree 2 poles (-19.3035, 5.9178) (-19.5426, 5.699) (-20.1504, 5.464) (-20.6082, 5.464) knots 0 0 0 1 2 2 2
  line L347 (-14.9843, 5.5532) -> (-18.477, 5.5532)
  line L348 (-18.477, 5.5532) -> (-18.477, 6.1731)
  line L349 (-18.477, 6.1731) -> (-15.8027, 9.9616)
  line L350 (-15.8027, 9.9616) -> (-18.3554, 9.9616)
  line L351 (-18.3554, 9.9616) -> (-18.3554, 10.5532)
  line L352 (-18.3554, 10.5532) -> (-15.0531, 10.5532)
  line L353 (-15.0531, 10.5532) -> (-15.0531, 9.9535)
  line L354 (-15.0531, 9.9535) -> (-17.7557, 6.1447)
  line L355 (-17.7557, 6.1447) -> (-14.9843, 6.1447)
  line L356 (-14.9843, 6.1447) -> (-14.9843, 5.5532)
  line L357 (-8.6026, 5.5532) -> (-9.3481, 5.5532)
  line L358 (-9.3481, 5.5532) -> (-11.5604, 9.8643)
  line L359 (-11.5604, 9.8643) -> (-11.5604, 5.5532)
  line L360 (-11.5604, 5.5532) -> (-12.1804, 5.5532)
  line L361 (-12.1804, 5.5532) -> (-12.1804, 10.5532)
  line L362 (-12.1804, 10.5532) -> (-11.2363, 10.5532)
  line L363 (-11.2363, 10.5532) -> (-9.2225, 6.5945)
  line L364 (-9.2225, 6.5945) -> (-9.2225, 10.5532)
  line L365 (-9.2225, 10.5532) -> (-8.6026, 10.5532)
  line L366 (-8.6026, 10.5532) -> (-8.6026, 5.5532)
  spline S124 degree 2 poles (-4.0523, 9.9818) (-3.7687, 9.6496) (-3.4527, 8.6771) (-3.4527, 8.0532) knots 0 0 0 1 2 2 2
  spline S125 degree 2 poles (-3.4527, 8.0532) (-3.4527, 7.4454) (-3.7606, 6.4608) (-4.0523, 6.1285) knots 0 0 0 1 2 2 2
  spline S126 degree 2 poles (-4.0523, 6.1285) (-4.3603, 5.7801) (-5.1747, 5.4478) (-5.665, 5.4478) knots 0 0 0 1 2 2 2
  spline S127 degree 2 poles (-5.665, 5.4478) (-6.1715, 5.4478) (-6.9818, 5.7922) (-7.2776, 6.1285) knots 0 0 0 1 2 2 2
  spline S128 degree 2 poles (-7.2776, 6.1285) (-7.5653, 6.4608) (-7.8732, 7.4373) (-7.8732, 8.0532) knots 0 0 0 1 2 2 2
  spline S129 degree 2 poles (-7.8732, 8.0532) (-7.8732, 8.6812) (-7.5612, 9.6374) (-7.2736, 9.9818) knots 0 0 0 1 2 2 2
  spline S130 degree 2 poles (-7.2736, 9.9818) (-6.9818, 10.3141) (-6.1674, 10.6585) (-5.665, 10.6585) knots 0 0 0 1 2 2 2
  spline S131 degree 2 poles (-5.665, 10.6585) (-5.1544, 10.6585) (-4.336, 10.3019) (-4.0523, 9.9818) knots 0 0 0 1 2 2 2
  spline S132 degree 2 poles (-4.1455, 8.0532) (-4.1455, 8.5475) (-4.3603, 9.3133) (-4.5548, 9.5645) knots 0 0 0 1 2 2 2
  spline S133 degree 2 poles (-4.5548, 9.5645) (-4.7533, 9.8238) (-5.3125, 10.0831) (-5.6609, 10.0831) knots 0 0 0 1 2 2 2
  spline S134 degree 2 poles (-5.6609, 10.0831) (-6.0215, 10.0831) (-6.5645, 9.8319) (-6.7711, 9.5645) knots 0 0 0 1 2 2 2
  spline S135 degree 2 poles (-6.7711, 9.5645) (-6.9697, 9.3092) (-7.1804, 8.5394) (-7.1804, 8.0532) knots 0 0 0 1 2 2 2
  spline S136 degree 2 poles (-7.1804, 8.0532) (-7.1804, 7.0686) (-6.3538, 6.0232) (-5.6609, 6.0232) knots 0 0 0 1 2 2 2
  spline S137 degree 2 poles (-5.6609, 6.0232) (-4.968, 6.0232) (-4.1455, 7.0686) (-4.1455, 8.0532) knots 0 0 0 1 2 2 2
  line L367 (2.8804, 10.5532) -> (1.6243, 5.5532)
  line L368 (1.6243, 5.5532) -> (0.8788, 5.5532)
  line L369 (0.8788, 5.5532) -> (-0.1382, 9.7023)
  line L370 (-0.1382, 9.7023) -> (-1.1269, 5.5532)
  line L371 (-1.1269, 5.5532) -> (-1.8643, 5.5532)
  line L372 (-1.8643, 5.5532) -> (-3.1407, 10.5532)
  line L373 (-3.1407, 10.5532) -> (-2.4559, 10.5532)
  line L374 (-2.4559, 10.5532) -> (-1.451, 6.4081)
  line L375 (-1.451, 6.4081) -> (-0.4543, 10.5532)
  line L376 (-0.4543, 10.5532) -> (0.2224, 10.5532)
  line L377 (0.2224, 10.5532) -> (1.2272, 6.3595)
  line L378 (1.2272, 6.3595) -> (2.2281, 10.5532)
  line L379 (2.2281, 10.5532) -> (2.8804, 10.5532)
  line L380 (2.9371, 5.5532) -> (4.6227, 10.5532)
  line L381 (4.6227, 10.5532) -> (5.4412, 10.5532)
  line L382 (5.4412, 10.5532) -> (7.1268, 5.5532)
  line L383 (7.1268, 5.5532) -> (6.4258, 5.5532)
  line L384 (6.4258, 5.5532) -> (5.972, 6.951)
  line L385 (5.972, 6.951) -> (4.0636, 6.951)
  line L386 (4.0636, 6.951) -> (3.6097, 5.5532)
  line L387 (3.6097, 5.5532) -> (2.9371, 5.5532)
  line L388 (5.7896, 7.5183) -> (5.0157, 9.8724)
  line L389 (5.0157, 9.8724) -> (4.2459, 7.5183)
  line L390 (4.2459, 7.5183) -> (5.7896, 7.5183)
  line L391 (11.4704, 5.5532) -> (10.6073, 5.5532)
  line L392 (10.6073, 5.5532) -> (9.0271, 7.5426)
  line L393 (9.0271, 7.5426) -> (8.2653, 7.5426)
  line L394 (8.2653, 7.5426) -> (8.2653, 5.5532)
  line L395 (8.2653, 5.5532) -> (7.6008, 5.5532)
  line L396 (7.6008, 5.5532) -> (7.6008, 10.5532)
  line L397 (7.6008, 10.5532) -> (8.8893, 10.5532)
  spline S138 degree 2 poles (8.8893, 10.5532) (9.3188, 10.5532) (9.8982, 10.46) (10.1616, 10.2898) knots 0 0 0 1 2 2 2
  spline S139 degree 2 poles (10.1616, 10.2898) (10.425, 10.1196) (10.7289, 9.5888) (10.7289, 9.1958) knots 0 0 0 1 2 2 2
  spline S140 degree 2 poles (10.7289, 9.1958) (10.7289, 8.6488) (10.1697, 7.9073) (9.6916, 7.729) knots 0 0 0 1 2 2 2
  line L398 (9.6916, 7.729) -> (11.4704, 5.5532)
  spline S141 degree 2 poles (10.036, 9.1431) (10.036, 9.3619) (9.882, 9.6982) (9.72, 9.8076) knots 0 0 0 1 2 2 2
  spline S142 degree 2 poles (9.72, 9.8076) (9.5781, 9.9008) (9.2013, 9.9778) (8.9258, 9.9778) knots 0 0 0 1 2 2 2
  line L399 (8.9258, 9.9778) -> (8.2653, 9.9778)
  line L400 (8.2653, 9.9778) -> (8.2653, 8.0977)
  line L401 (8.2653, 8.0977) -> (8.8488, 8.0977)
  spline S143 degree 2 poles (8.8488, 8.0977) (9.1365, 8.0977) (9.5943, 8.199) (9.7524, 8.357) knots 0 0 0 1 2 2 2
  spline S144 degree 2 poles (9.7524, 8.357) (9.8982, 8.4948) (10.036, 8.8838) (10.036, 9.1431) knots 0 0 0 1 2 2 2
  line L402 (15.5141, 5.5532) -> (14.6511, 5.5532)
  line L403 (14.6511, 5.5532) -> (12.8237, 7.8789)
  line L404 (12.8237, 7.8789) -> (12.532, 7.5507)
  line L405 (12.532, 7.5507) -> (12.532, 5.5532)
  line L406 (12.532, 5.5532) -> (11.8674, 5.5532)
  line L407 (11.8674, 5.5532) -> (11.8674, 10.5532)
  line L408 (11.8674, 10.5532) -> (12.532, 10.5532)
  line L409 (12.532, 10.5532) -> (12.532, 8.2557)
  line L410 (12.532, 8.2557) -> (14.5822, 10.5532)
  line L411 (14.5822, 10.5532) -> (15.3926, 10.5532)
  line L412 (15.3926, 10.5532) -> (13.3221, 8.3206)
  line L413 (13.3221, 8.3206) -> (15.5141, 5.5532)
  line L414 (17.6535, 5.5532) -> (15.7167, 5.5532)
  line L415 (15.7167, 5.5532) -> (15.7167, 6.0637)
  line L416 (15.7167, 6.0637) -> (16.3529, 6.0637)
  line L417 (16.3529, 6.0637) -> (16.3529, 10.0426)
  line L418 (16.3529, 10.0426) -> (15.7167, 10.0426)
  line L419 (15.7167, 10.0426) -> (15.7167, 10.5532)
  line L420 (15.7167, 10.5532) -> (17.6535, 10.5532)
  line L421 (17.6535, 10.5532) -> (17.6535, 10.0426)
  line L422 (17.6535, 10.0426) -> (17.0174, 10.0426)
  line L423 (17.0174, 10.0426) -> (17.0174, 6.0637)
  line L424 (17.0174, 6.0637) -> (17.6535, 6.0637)
  line L425 (17.6535, 6.0637) -> (17.6535, 5.5532)
  line L426 (18.476, 5.5532) -> (18.476, 10.5532)
  line L427 (18.476, 10.5532) -> (21.6041, 10.5532)
  line L428 (21.6041, 10.5532) -> (21.6041, 9.9616)
  line L429 (21.6041, 9.9616) -> (19.1405, 9.9616)
  line L430 (19.1405, 9.9616) -> (19.1405, 8.5921)
  line L431 (19.1405, 8.5921) -> (21.4379, 8.5921)
  line L432 (21.4379, 8.5921) -> (21.4379, 8.0005)
  line L433 (21.4379, 8.0005) -> (19.1405, 8.0005)
  line L434 (19.1405, 8.0005) -> (19.1405, 6.1447)
  line L435 (19.1405, 6.1447) -> (21.6041, 6.1447)
  line L436 (21.6041, 6.1447) -> (21.6041, 5.5532)
  line L437 (21.6041, 5.5532) -> (18.476, 5.5532)
  line L438 (27.9371, 10.5532) -> (26.6811, 5.5532)
  line L439 (26.6811, 5.5532) -> (25.9355, 5.5532)
  line L440 (25.9355, 5.5532) -> (24.9185, 9.7023)
  line L441 (24.9185, 9.7023) -> (23.9298, 5.5532)
  line L442 (23.9298, 5.5532) -> (23.1924, 5.5532)
  line L443 (23.1924, 5.5532) -> (21.9161, 10.5532)
  line L444 (21.9161, 10.5532) -> (22.6008, 10.5532)
  line L445 (22.6008, 10.5532) -> (23.6057, 6.4081)
  line L446 (23.6057, 6.4081) -> (24.6025, 10.5532)
  line L447 (24.6025, 10.5532) -> (25.2791, 10.5532)
  line L448 (25.2791, 10.5532) -> (26.284, 6.3595)
  line L449 (26.284, 6.3595) -> (27.2848, 10.5532)
  line L450 (27.2848, 10.5532) -> (27.9371, 10.5532)
  line L451 (30.2751, 5.5532) -> (28.3383, 5.5532)
  line L452 (28.3383, 5.5532) -> (28.3383, 6.0637)
  line L453 (28.3383, 6.0637) -> (28.9744, 6.0637)
  line L454 (28.9744, 6.0637) -> (28.9744, 10.0426)
  line L455 (28.9744, 10.0426) -> (28.3383, 10.0426)
  line L456 (28.3383, 10.0426) -> (28.3383, 10.5532)
  line L457 (28.3383, 10.5532) -> (30.2751, 10.5532)
  line L458 (30.2751, 10.5532) -> (30.2751, 10.0426)
  line L459 (30.2751, 10.0426) -> (29.6389, 10.0426)
  line L460 (29.6389, 10.0426) -> (29.6389, 6.0637)
  line L461 (29.6389, 6.0637) -> (30.2751, 6.0637)
  line L462 (30.2751, 6.0637) -> (30.2751, 5.5532)
  spline S145 degree 2 poles (33.0506, 5.464) (32.5644, 5.464) (31.7418, 5.7922) (31.442, 6.1204) knots 0 0 0 1 2 2 2
  spline S146 degree 2 poles (31.442, 6.1204) (31.1422, 6.4446) (30.814, 7.417) (30.814, 8.0491) knots 0 0 0 1 2 2 2
  spline S147 degree 2 poles (30.814, 8.0491) (30.814, 8.6771) (31.1341, 9.6091) (31.4379, 9.9535) knots 0 0 0 1 2 2 2
  spline S148 degree 2 poles (31.4379, 9.9535) (31.7378, 10.2898) (32.5563, 10.6423) (33.0627, 10.6423) knots 0 0 0 1 2 2 2
  spline S149 degree 2 poles (33.0627, 10.6423) (33.314, 10.6423) (33.7556, 10.5694) (33.942, 10.5126) knots 0 0 0 1 2 2 2
  spline S150 degree 2 poles (33.942, 10.5126) (34.1041, 10.46) (34.4404, 10.31) (34.6065, 10.2209) knots 0 0 0 1 2 2 2
  line L463 (34.6065, 10.2209) -> (34.6065, 9.4186)
  line L464 (34.6065, 9.4186) -> (34.5538, 9.4186)
  spline S151 degree 2 poles (34.5538, 9.4186) (34.4647, 9.4997) (34.1892, 9.7266) (33.9906, 9.836) knots 0 0 0 1 2 2 2
  spline S152 degree 2 poles (33.9906, 9.836) (33.8002, 9.9413) (33.3504, 10.075) (33.0587, 10.075) knots 0 0 0 1 2 2 2
  spline S153 degree 2 poles (33.0587, 10.075) (32.7386, 10.075) (32.1673, 9.8117) (31.9525, 9.5604) knots 0 0 0 1 2 2 2
  spline S154 degree 2 poles (31.9525, 9.5604) (31.7418, 9.3052) (31.5068, 8.5313) (31.5068, 8.0491) knots 0 0 0 1 2 2 2
  spline S155 degree 2 poles (31.5068, 8.0491) (31.5068, 7.5345) (31.754, 6.793) (31.9687, 6.5378) knots 0 0 0 1 2 2 2
  spline S156 degree 2 poles (31.9687, 6.5378) (32.1794, 6.2906) (32.7426, 6.0394) (33.0587, 6.0394) knots 0 0 0 1 2 2 2
  spline S157 degree 2 poles (33.0587, 6.0394) (33.3464, 6.0394) (33.8367, 6.1812) (34.0271, 6.2865) knots 0 0 0 1 2 2 2
  spline S158 degree 2 poles (34.0271, 6.2865) (34.2094, 6.3919) (34.4809, 6.6107) (34.5579, 6.6877) knots 0 0 0 1 2 2 2
  line L465 (34.5579, 6.6877) -> (34.6065, 6.6877)
  line L466 (34.6065, 6.6877) -> (34.6065, 5.8935)
  spline S159 degree 2 poles (34.6065, 5.8935) (34.4404, 5.8165) (34.1486, 5.6747) (33.942, 5.6099) knots 0 0 0 1 2 2 2
  spline S160 degree 2 poles (33.942, 5.6099) (33.7232, 5.5369) (33.3504, 5.464) (33.0506, 5.464) knots 0 0 0 1 2 2 2
  line L467 (38.4153, 5.5532) -> (34.9225, 5.5532)
  line L468 (34.9225, 5.5532) -> (34.9225, 6.1731)
  line L469 (34.9225, 6.1731) -> (37.5968, 9.9616)
  line L470 (37.5968, 9.9616) -> (35.0441, 9.9616)
  line L471 (35.0441, 9.9616) -> (35.0441, 10.5532)
  line L472 (35.0441, 10.5532) -> (38.3464, 10.5532)
  line L473 (38.3464, 10.5532) -> (38.3464, 9.9535)
  line L474 (38.3464, 9.9535) -> (35.6438, 6.1447)
  line L475 (35.6438, 6.1447) -> (38.4153, 6.1447)
  line L476 (38.4153, 6.1447) -> (38.4153, 5.5532)
  spline S161 degree 2 poles (-39.0625, 0.8135) (-39.0625, 0.4893) (-39.2934, -0.0941) (-39.5001, -0.2967) knots 0 0 0 1 2 2 2
  spline S162 degree 2 poles (-39.5001, -0.2967) (-39.7594, -0.552) (-40.4604, -0.8154) (-40.9952, -0.8154) knots 0 0 0 1 2 2 2
  line L477 (-40.9952, -0.8154) -> (-41.5584, -0.8154)
  line L478 (-41.5584, -0.8154) -> (-41.5584, -2.6792)
  line L479 (-41.5584, -2.6792) -> (-42.2229, -2.6792)
  line L480 (-42.2229, -2.6792) -> (-42.2229, 2.3208)
  line L481 (-42.2229, 2.3208) -> (-40.9668, 2.3208)
  spline S163 degree 2 poles (-40.9668, 2.3208) (-40.5211, 2.3208) (-39.8971, 2.1749) (-39.6581, 2.0088) knots 0 0 0 1 2 2 2
  spline S164 degree 2 poles (-39.6581, 2.0088) (-39.3785, 1.8184) (-39.0625, 1.2308) (-39.0625, 0.8135) knots 0 0 0 1 2 2 2
  spline S165 degree 2 poles (-39.7553, 0.7932) (-39.7553, 1.0526) (-39.9336, 1.4334) (-40.1159, 1.555) knots 0 0 0 1 2 2 2
  spline S166 degree 2 poles (-40.1159, 1.555) (-40.274, 1.6603) (-40.6954, 1.7454) (-41.0074, 1.7454) knots 0 0 0 1 2 2 2
  line L482 (-41.0074, 1.7454) -> (-41.5584, 1.7454)
  line L483 (-41.5584, 1.7454) -> (-41.5584, -0.2481)
  line L484 (-41.5584, -0.2481) -> (-41.1046, -0.2481)
  spline S167 degree 2 poles (-41.1046, -0.2481) (-40.6994, -0.2481) (-40.201, -0.1184) (-40.039, 0.0517) knots 0 0 0 1 2 2 2
  spline S168 degree 2 poles (-40.039, 0.0517) (-39.889, 0.2017) (-39.7553, 0.5542) (-39.7553, 0.7932) knots 0 0 0 1 2 2 2
  spline S169 degree 2 poles (-34.8931, 1.7495) (-34.6095, 1.4172) (-34.2934, 0.4448) (-34.2934, -0.1792) knots 0 0 0 1 2 2 2
  spline S170 degree 2 poles (-34.2934, -0.1792) (-34.2934, -0.787) (-34.6014, -1.7716) (-34.8931, -2.1038) knots 0 0 0 1 2 2 2
  spline S171 degree 2 poles (-34.8931, -2.1038) (-35.201, -2.4523) (-36.0155, -2.7846) (-36.5057, -2.7846) knots 0 0 0 1 2 2 2
  spline S172 degree 2 poles (-36.5057, -2.7846) (-37.0122, -2.7846) (-37.8226, -2.4402) (-38.1184, -2.1038) knots 0 0 0 1 2 2 2
  spline S173 degree 2 poles (-38.1184, -2.1038) (-38.4061, -1.7716) (-38.714, -0.7951) (-38.714, -0.1792) knots 0 0 0 1 2 2 2
  spline S174 degree 2 poles (-38.714, -0.1792) (-38.714, 0.4488) (-38.402, 1.4051) (-38.1143, 1.7495) knots 0 0 0 1 2 2 2
  spline S175 degree 2 poles (-38.1143, 1.7495) (-37.8226, 2.0817) (-37.0082, 2.4261) (-36.5057, 2.4261) knots 0 0 0 1 2 2 2
  spline S176 degree 2 poles (-36.5057, 2.4261) (-35.9952, 2.4261) (-35.1767, 2.0696) (-34.8931, 1.7495) knots 0 0 0 1 2 2 2
  spline S177 degree 2 poles (-34.9863, -0.1792) (-34.9863, 0.3151) (-35.201, 1.0809) (-35.3955, 1.3321) knots 0 0 0 1 2 2 2
  spline S178 degree 2 poles (-35.3955, 1.3321) (-35.5941, 1.5915) (-36.1532, 1.8508) (-36.5017, 1.8508) knots 0 0 0 1 2 2 2
  spline S179 degree 2 poles (-36.5017, 1.8508) (-36.8623, 1.8508) (-37.4052, 1.5996) (-37.6119, 1.3321) knots 0 0 0 1 2 2 2
  spline S180 degree 2 poles (-37.6119, 1.3321) (-37.8104, 1.0769) (-38.0211, 0.307) (-38.0211, -0.1792) knots 0 0 0 1 2 2 2
  spline S181 degree 2 poles (-38.0211, -0.1792) (-38.0211, -1.1638) (-37.1946, -2.2092) (-36.5017, -2.2092) knots 0 0 0 1 2 2 2
  spline S182 degree 2 poles (-36.5017, -2.2092) (-35.8088, -2.2092) (-34.9863, -1.1638) (-34.9863, -0.1792) knots 0 0 0 1 2 2 2
  spline S183 degree 2 poles (-29.6216, -0.1833) (-29.6216, -0.868) (-30.1767, -1.9701) (-30.6427, -2.2781) knots 0 0 0 1 2 2 2
  spline S184 degree 2 poles (-30.6427, -2.2781) (-31.0236, -2.5171) (-31.8056, -2.6792) (-32.4134, -2.6792) knots 0 0 0 1 2 2 2
  line L485 (-32.4134, -2.6792) -> (-33.5641, -2.6792)
  line L486 (-33.5641, -2.6792) -> (-33.5641, 2.3208)
  line L487 (-33.5641, 2.3208) -> (-32.4255, 2.3208)
  spline S185 degree 2 poles (-32.4255, 2.3208) (-31.7205, 2.3208) (-30.9182, 2.1101) (-30.6346, 1.9237) knots 0 0 0 1 2 2 2
  spline S186 degree 2 poles (-30.6346, 1.9237) (-30.1524, 1.6036) (-29.6216, 0.5461) (-29.6216, -0.1833) knots 0 0 0 1 2 2 2